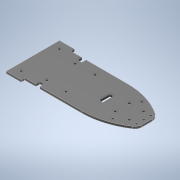
# Autodesk Inventor part: body
Saved by Autodesk Inventor 2022 (Build 260153000, 153)
## iProperties
Created: 2021-07-05
Part Number: body
Material: アクリル
Document SubType Name: Modeling
Designer: ken
Density: 1.188 g/cm^3
Appearance: 滑らか - 黒
Mass: 34.3362 g
Surface Area: 212.301 cm^2
Volume: 28.9025 cm^3
Author: ken
Autodesk Inventor part; units mm, degrees
ref_plane "YZ Plane" through (0, 0, 0) normal (1, 0, 0) x (0, 1, 0)
ref_plane "XZ Plane" through (0, 0, 0) normal (0, 1, 0) x (-1, 0, 0)
ref_plane "XY Plane" through (0, 0, 0) normal (0, 0, 1) x (1, 0, 0)
sketch "スケッチ1" plane through (0, 0, 0) normal (0, 1, 0) x (-1, 0, 0)
  line L0 (0, 0) -> (140, 0)
  line L1 (140, -65) -> (0, -65)
  line L2 (0, -65) -> (0, 0)
  line L3 (124.5, 0) -> (118.5, 0)
  line L4 (118.5, 0) -> (118.5, -6)
  line L5 (118.5, -6) -> (124.5, -6)
  line L6 (124.5, -6) -> (124.5, 0)
  line L7 (124.5, -65) -> (118.5, -65)
  line L8 (118.5, -65) -> (118.5, -59)
  line L9 (118.5, -59) -> (124.5, -59)
  line L10 (124.5, -59) -> (124.5, -65)
  line L11 (0, -45) -> (25, -65)
  line L12 (0, -20) -> (25, 0)
  line L13 (60, -25) -> (55, -25)
  line L14 (55, -25) -> (55, -40)
  line L15 (55, -40) -> (60, -40)
  line L16 (60, -40) -> (60, -25)
  line L17 (140, -70) -> (161, -70)
  line L18 (161, -70) -> (161, 5)
  line L19 (161, 5) -> (140, 5)
  line L20 (140, -65) -> (140, -70)
  line L21 (140, 0) -> (140, 5)
  point P0 (124.5, -3)
  point P1 (124.5, -62)
  point P2 (118.5, 0)
  dimension "d0" = 140
  dimension "d1" = 65
  dimension "d61" = 6
  dimension "d62" = 6
  dimension "d63" = 6
  dimension "d64" = 6
  dimension "d66" = 20
  dimension "d67" = 20
  dimension "d68" = 25
  dimension "d70" = 5
  dimension "d71" = 15
  dimension "d73" = 25
  dimension "d103" = 21
  dimension "d104" = 75
  dimension "d105" = 5
  constraints: 44 end point, 9 equal length, 6 point on line, 5 horizontal, 4 perpendicular, 2 midpoint, 2 vertical alignment, 1 vertical
  measures "d0" distance of L1.start L1.end
  measures "d1" distance of L0.end L1.start
  measures "d61" distance of L5.end L4.end
  measures "d62" distance of L4.end L3.end
  measures "d63" distance of L8.end L9.end
  measures "d64" distance of L7.end L8.end
  measures "d66" distance of L0.start L12.start
  measures "d67" distance of L1.end L11.start
  measures "d68" distance of L0.start L12.end
  measures "d70" distance of L15.end L14.end
  measures "d71" distance of L14.end L13.end
  measures "d73" distance between parallel lines of L0 L13
  measures "d103" distance of L19.end L18.end
  measures "d104" distance of L18.end L17.end
  measures "d105" distance between parallel lines of L17 L1
extrude "押し出し1" add sketch "スケッチ1" along normal blind 3 contours L0 L4 L5 L6 L21 L19 L18 L17 L20 L1 L10 L9 L8 L11 L2 L12
sketch "スケッチ2" plane through (0, 3, 0) normal (0, 1, 0) x (1, 0, 0)
  line L0 (-140, 0) -> (0, 0) projected
  line L1 (-25, 65) -> (-140, 65) projected
  line L2 (-140, 65) -> (-140, 70) projected
  point P0 (-121.5, 12.5)
  point P1 (0, 65)
  point P2 (-121.5, 52.5)
  dimension "d9" = 12.5
  dimension "d55" = 12.5
  dimension "d69" = 40
  dimension "d107" = 18.5
  measures "d9" distance from line of L0 point (-121.5, 12.5)
  measures "d55" distance from line of L1 point (-121.5, 52.5)
  measures "d69" distance of point (-121.5, 12.5) point (-121.5, 52.5)
  measures "d107" distance from line of L2 point (-121.5, 52.5)
hole "穴1" at (-121.5, 3, -12.5) at (-121.5, 3, -52.5) direction (0, -1, 0) diameter 3.2 end through all
sketch "スケッチ3" plane through (0, 3, 0) normal (0, 1, 0) x (1, 0, 0)
  line L0 (-140, 0) -> (0, 0) projected
  line L1 (-25, 65) -> (-140, 65) projected
  line L2 (0, 0) -> (0, 45) projected
  point P0 (-35, 22.5)
  point P1 (-35, 42.5)
  point P2 (-15, 42.5)
  point P3 (-15, 22.5)
  point P4 (0, 65)
  dimension "d20" = 20
  dimension "d21" = 20
  dimension "d22" = 22.5
  dimension "d24" = 15
  constraints: 2 horizontal alignment, 2 vertical alignment
  measures "d20" distance of point (-35, 42.5) point (-35, 22.5)
  measures "d21" distance of point (-15, 42.5) point (-35, 42.5)
  measures "d22" distance from line of L0 point (-35, 22.5)
  measures "d24" distance from line of L2 point (-15, 42.5)
hole "穴2" at (-35, 3, -22.5) at (-35, 3, -42.5) at (-15, 3, -42.5) at (-15, 3, -22.5) direction (0, -1, 0) diameter 3.2 end through all
sketch "スケッチ4" plane through (0, 3, 0) normal (0, 1, 0) x (1, 0, 0)
  line L0 (-25, 65) -> (-140, 65) projected
  line L1 (0, 0) -> (0, 45) projected
  point P0 (-5, 42.5)
  point P1 (-5, 32.5)
  point P2 (-5, 22.5)
  point P3 (0, 65)
  dimension "d32" = 10
  dimension "d33" = 10
  dimension "d34" = 32.5
  dimension "d35" = 5
  constraints: 2 vertical alignment
  measures "d32" distance of point (-5, 42.5) point (-5, 32.5)
  measures "d33" distance of point (-5, 22.5) point (-5, 32.5)
  measures "d34" distance from line of L0 point (-5, 32.5)
  measures "d35" distance from line of L1 point (-5, 42.5)
hole "穴3" at (-5, 3, -42.5) at (-5, 3, -32.5) at (-5, 3, -22.5) direction (0, -1, 0) diameter 3.2 end through all
sketch "スケッチ5" plane through (0, 3, 0) normal (0, 1, 0) x (1, 0, 0)
  line L0 (-25, 65) -> (-140, 65) projected
  line L1 (-140, 65) -> (-140, 0) projected
  line L2 (-140, 65) -> (-140, 70) projected
  point P0 (0, 0)
  point P1 (-94, 53)
  point P2 (-28, 53)
  point P3 (-28, 12)
  point P4 (-94, 12)
  point P5 (0, 65)
  dimension "d43" = 66
  dimension "d44" = 41
  dimension "d46" = 12
  dimension "d106" = 46
  constraints: 2 horizontal alignment, 2 vertical alignment
  measures "d43" distance of point (-94, 53) point (-28, 53)
  measures "d44" distance of point (-94, 12) point (-94, 53)
  measures "d46" distance from line of L0 point (-94, 53)
  measures "d106" distance from line of L2 point (-94, 53)
hole "穴4" at (-94, 3, -53) at (-28, 3, -53) at (-28, 3, -12) at (-94, 3, -12) direction (0, -1, 0) diameter 3.2 end through all
sketch "スケッチ8" plane through (0, 3, 0) normal (0, 1, 0) x (1, 0, 0)
  line L0 (-140, 70) -> (-161, 70) projected
  line L1 (-161, 70) -> (-161, -5) projected
  point P0 (0, 0)
  point P1 (-150.5, 59.35)
  point P2 (-150.5, 5.65)
  dimension "d108" = 10.65
  dimension "d109" = 10.5
  dimension "d110" = 53.7
  constraints: 1 vertical alignment
  measures "d108" distance from line of L0 point (-150.5, 59.35)
  measures "d109" distance from line of L1 point (-150.5, 59.35)
  measures "d110" distance of point (-150.5, 5.65) point (-150.5, 59.35)
hole "穴5" at (-150.5, 3, -59.35) at (-150.5, 3, -5.65) direction (0, -1, 0) diameter 3.2 end through all
sketch "スケッチ7" plane through (0, 3, 0) normal (0, 1, 0) x (1, 0, 0)
  line L0 (-140, 65) -> (-124.5, 65)
  line L1 (-124.5, 59) -> (-124.5, 65) projected
  line L2 (-124.5, 65) -> (-124.5, 59)
  line L3 (-118.5, 59) -> (-124.5, 59) projected
  line L4 (-124.5, 59) -> (-118.5, 59)
  line L5 (-118.5, 65) -> (-118.5, 59) projected
  line L6 (-118.5, 59) -> (-118.5, 65)
  line L7 (-118.5, 65) -> (-60.0781, 65)
  line L8 (0, 39.7809) -> (0, 25.2191)
  line L9 (-60.0781, 0) -> (-118.5, 0)
  line L10 (-118.5, 0) -> (-118.5, 6)
  line L11 (-118.5, 6) -> (-124.5, 6)
  line L12 (-124.5, 6) -> (-124.5, 0)
  line L13 (-124.5, 0) -> (-140, 0)
  circle A0 centre (-121.5, 52.5) radius 1.6
  circle A1 centre (-121.5, 12.5) radius 1.6
  line L14 (-60, 40) -> (-55, 40) projected
  line L15 (-55, 40) -> (-55, 25) projected
  line L16 (-60, 40) -> (-55, 40)
  line L17 (-55, 40) -> (-55, 25)
  line L18 (-55, 25) -> (-60, 25)
  line L19 (-60, 25) -> (-60, 40)
  circle A2 centre (-94, 53) radius 1.6
  circle A3 centre (-94, 12) radius 1.6
  circle A4 centre (-28, 53) radius 1.6
  circle A5 centre (-28, 12) radius 1.6
  circle A6 centre (-35, 42.5) radius 1.6
  circle A7 centre (-15, 42.5) radius 1.6
  circle A8 centre (-35, 22.5) radius 1.6
  circle A9 centre (-15, 22.5) radius 1.6
  circle A10 centre (-5, 42.5) radius 1.6
  circle A11 centre (-5, 32.5) radius 1.6
  circle A12 centre (-5, 22.5) radius 1.6
  line L20 (-140, 65) -> (-140, 70)
  line L21 (-140, 70) -> (-161, 70) projected
  line L22 (-140, 70) -> (-161, 70)
  line L23 (-161, 70) -> (-161, -5) projected
  line L24 (-161, 70) -> (-161, -5)
  line L25 (-161, -5) -> (-140, -5) projected
  line L26 (-161, -5) -> (-140, -5)
  line L27 (-140, -5) -> (-140, 0) projected
  line L28 (-140, -5) -> (-140, 0)
  circle A13 centre (-150.5, 59.35) radius 1.6 projected
  circle A14 centre (-150.5, 59.35) radius 1.6
  circle A15 centre (-150.5, 5.65) radius 1.6
  arc A16 (-60.0781, 0) -> (-4.4358, 16.9101) centre (-60.0781, 100) ccw
  arc A17 (-4.4358, 48.0899) -> (-60.0781, 65) centre (-60.0781, -35) ccw
  arc A18 (0, 39.7809) -> (-4.4358, 48.0899) centre (-10, 39.7809) ccw
  arc A19 (-4.4358, 16.9101) -> (0, 25.2191) centre (-10, 25.2191) ccw
  point P0 (0, 0)
  point P1 (-25, 65)
  point P2 (0, 45)
  point P3 (-25, 0)
  point P4 (0, 20)
  dimension "d74" = 3.2
  dimension "d75" = 3.2
  dimension "d77" = 40
  dimension "d79" = 3.2
  dimension "d80" = 3.2
  dimension "d81" = 3.2
  dimension "d82" = 3.2
  dimension "d83" = 41
  dimension "d86" = 66
  dimension "d87" = 3.2
  dimension "d88" = 3.2
  dimension "d89" = 3.2
  dimension "d90" = 3.2
  dimension "d91" = 20
  dimension "d92" = 20
  dimension "d94" = 15
  dimension "d95" = 3.2
  dimension "d96" = 3.2
  dimension "d97" = 3.2
  dimension "d98" = 10
  dimension "d99" = 10
  dimension "d100" = 5
  dimension "d118" = 18.5
  dimension "d119" = 46
  dimension "d121" = 161
  dimension "d123" = 3.2
  dimension "d124" = 3.2
  dimension "d125" = 10.5
  dimension "d126" = 10.65
  dimension "d127" = 53.7
  dimension "d129" = 6
  dimension "d133" = 100
  dimension "d134" = 10
  dimension "d138" = 32.5
  dimension "d139" = 22.5
  dimension "d140" = 12
  dimension "d141" = 16.9101
  dimension "d142" = 16.9101
  constraints: 40 end point, 19 centre point, 12 perpendicular, 9 vertical alignment, 8 point on circle, 6 tangent, 4 horizontal alignment, 4 parallel, 4 point on line, 2 equal radius, 1 coincident, 1 horizontal, 1 vertical
  measures "d74" diameter of A0
  measures "d75" diameter of A1
  measures "d77" distance of A0.centre A1.centre
  measures "d79" diameter of A2
  measures "d80" diameter of A3
  measures "d81" diameter of A4
  measures "d82" diameter of A5
  measures "d83" distance of A3.centre A2.centre
  measures "d86" distance of A2.centre A4.centre
  measures "d87" diameter of A6
  measures "d88" diameter of A7
  measures "d89" diameter of A8
  measures "d90" diameter of A9
  measures "d91" distance of A6.centre A7.centre
  measures "d92" distance of A8.centre A6.centre
  measures "d94" distance from line of L8 A7.centre
  measures "d95" diameter of A10
  measures "d96" diameter of A11
  measures "d97" diameter of A12
  measures "d98" distance of A11.centre A10.centre
  measures "d99" distance of A12.centre A11.centre
  measures "d100" distance from line of L8 A10.centre
  measures "d118" distance from line of L20 A0.centre
  measures "d119" distance from line of L20 A2.centre
  measures "d121" distance between parallel lines of L8 L23
  measures "d123" diameter of A14
  measures "d124" diameter of A15
  measures "d125" distance from line of L24 A14.centre
  measures "d126" distance from line of L21 A13.centre
  measures "d127" distance of A15.centre A13.centre
  measures "d129" distance between parallel lines of L10 L12
  measures "d133" radius of A16
  measures "d134" radius of A18
  measures "d138" distance from line of A11.centre L7
  measures "d139" distance from line of L7 A6.centre
  measures "d140" distance from line of L7 A4.centre
  measures "d141" distance from line of L9 A16.end
  measures "d142" distance from line of L7 A17.start
fillet "フィレット1" radius 100 1 edges at (-25, 1.5, 0)
fillet "フィレット2" radius 100 1 edges at (-25, 1.5, -65)
fillet "フィレット3" radius 10 1 edges at (0, 1.5, -20)
fillet "フィレット4" radius 10 1 edges at (0, 1.5, -45)
